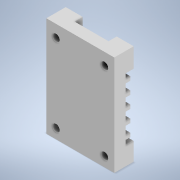
# Autodesk Inventor part: Belt Clamp
Saved by Autodesk Inventor 2020 (Build 240168000, 168)
## iProperties
Created: 2020-03-18
Part Number: Belt Clamp
Material: Generic
Document SubType Name: Modeling
Designer: DasNick
Density: 1 g/cm^3
Appearance: Default
Author: DasNick
Autodesk Inventor part; units mm, degrees
ref_plane "YZ Plane" through (0, 0, 0) normal (1, 0, 0) x (0, 1, 0)
ref_plane "XZ Plane" through (0, 0, 0) normal (0, 1, 0) x (-1, 0, 0)
sketch "Sketch1" plane through (0, 0, 0) normal (0, 0, 1) x (1, 0, 0)
  circle A0 centre (22.3624, 24.7247) radius 2.3813 projected
  circle A1 centre (22.3624, -26.3473) radius 2.3813 projected
  circle A2 centre (-9.3876, 24.7247) radius 2.3813 projected
  circle A3 centre (-9.3876, -26.3473) radius 2.3813 projected
  line L0 (28.7124, 32.6973) -> (-15.7376, 32.6973) projected
  line L1 (-15.7376, 32.6973) -> (-15.7376, -32.6973) projected
  line L2 (-15.7376, -32.6973) -> (28.7124, -32.6973) projected
  line L3 (28.7124, -32.6973) -> (28.7124, 32.6973) projected
  point P0 (0, 0)
extrude "Extrusion1" add sketch "Sketch1" along normal blind 12.7
sketch "Sketch2" plane through (-15.7376, -32.6973, 0) normal (0, -1, 0) x (1, 0, 0)
  line L0 (11.1075, 69.4178) -> (11.1075, 0)
  line L1 (33.3375, 69.1638) -> (33.3375, 0)
  line L2 (11.1075, 0) -> (33.3375, 0)
  line L3 (0, 9.525) -> (44.45, 9.525)
  line L4 (11.1075, 0) -> (33.3375, 0)
  line L5 (33.3375, 0) -> (33.3375, 5.334)
  line L6 (33.3375, 5.334) -> (11.1075, 5.334)
  line L7 (11.1075, 5.334) -> (11.1075, 0)
  line L8 (0, 0) -> (44.45, 0) projected
  point P0 (15.875, 0)
  point P1 (11.1075, 5.334)
  dimension "d2" = 5.334
  dimension "d21" = 0
  constraints: 16 end point, 1 point on line
  measures "d2" distance of L5.end L4.end
  measures "d21" distance between parallel lines of L8 L2
extrude "Extrusion2" cut sketch "Sketch2" against normal blind 76.2 contours L6 L1 L2 L0
ref_plane "Work Plane1" through (-16.0653, -32.8267, -33.655) normal (0, 0, -1) x (0, 1, 0)
sketch "Sketch3" plane through (17.5999, -32.6973, 5.334) normal (0, 0, -1) x (-1, 0, 0)
  line L0 (0, 0) -> (0, 65.3946) projected
  line L1 (0, 46.9796) -> (22.23, 46.9796)
  line L2 (22.23, 46.9796) -> (22.23, 49.5196)
  line L3 (22.23, 49.5196) -> (0, 49.5196)
  line L4 (0, 49.5196) -> (0, 46.9796)
  line L5 (0, 65.3946) -> (22.23, 65.3946) projected
  line L6 (33.3375, 65.3946) -> (33.3375, 0) projected
  line L7 (0, 38.9796) -> (22.23, 38.9796)
  line L8 (22.23, 38.9796) -> (22.23, 41.5196)
  line L9 (22.23, 41.5196) -> (0, 41.5196)
  line L10 (0, 41.5196) -> (0, 38.9796)
  line L11 (0, 30.9796) -> (22.23, 30.9796)
  line L12 (22.23, 30.9796) -> (22.23, 33.5196)
  line L13 (22.23, 33.5196) -> (0, 33.5196)
  line L14 (0, 33.5196) -> (0, 30.9796)
  line L15 (0, 22.9796) -> (22.23, 22.9796)
  line L16 (22.23, 22.9796) -> (22.23, 25.5196)
  line L17 (22.23, 25.5196) -> (0, 25.5196)
  line L18 (0, 25.5196) -> (0, 22.9796)
  line L19 (0, 14.9796) -> (22.23, 14.9796)
  line L20 (22.23, 14.9796) -> (22.23, 17.5196)
  line L21 (22.23, 17.5196) -> (0, 17.5196)
  line L22 (0, 17.5196) -> (0, 14.9796)
  point P0 (17.5999, 32.6973)
  point P1 (0, 17.5196)
  point P2 (0, 14.9796)
  point P3 (0, 25.5196)
  point P4 (0, 22.9796)
  point P5 (0, 33.5196)
  point P6 (0, 30.9796)
  point P7 (0, 41.5196)
  point P8 (0, 38.9796)
  point P9 (0, 49.5196)
  dimension "d6" = 15.875
  dimension "d7" = 2.54
  dimension "d10" = 8
  constraints: 40 end point, 2 parallel, 1 horizontal, 1 perpendicular, 1 point on line, 1 vertical, 32 other
  measures "d6" distance between parallel lines of L5 L3
  measures "d7" distance between parallel lines of L3 L1
  measures "d10" distance of L1.start L7.start
extrude "Extrusion3" add sketch "Sketch3" along normal blind 5.334
sketch "Sketch4" plane through (0, 0, 0) normal (0, 0, -1) x (-1, 0, 0)
  line L0 (4.6301, 14.2823) -> (4.6301, 16.8223)
  line L1 (15.7376, 32.6973) -> (15.7376, -32.6973) projected
  line L2 (4.6301, 16.8223) -> (15.7376, 16.8223)
  line L3 (15.7376, 16.8223) -> (15.7376, 19.9973)
  line L4 (15.7376, 19.9973) -> (4.6301, 19.9973)
  line L5 (4.6301, 19.9973) -> (4.6301, 16.8223)
  line L6 (4.6301, 14.2823) -> (4.6301, 8.8223)
  line L7 (4.6301, 6.2823) -> (4.6301, 0.8223)
  line L8 (4.6301, -1.7177) -> (4.6301, -7.1777)
  line L9 (4.6301, -9.7177) -> (4.6301, -15.1777)
  line L10 (-17.5999, 14.2823) -> (4.6301, 14.2823)
  line L11 (4.6301, 14.2823) -> (15.7376, 14.2823)
  line L12 (15.7376, 14.2823) -> (15.7376, 8.8223)
  line L13 (15.7376, 8.8223) -> (4.6301, 8.8223)
  line L14 (4.6301, 8.8223) -> (4.6301, 14.2823)
  line L15 (4.6301, 0.8223) -> (4.6301, 6.2823)
  line L16 (4.6301, 6.2823) -> (15.7376, 6.2823)
  line L17 (15.7376, 6.2823) -> (15.7376, 0.8223)
  line L18 (15.7376, 0.8223) -> (4.6301, 0.8223)
  line L19 (4.6301, 0.8223) -> (4.6301, 6.2823)
  line L20 (4.6301, -7.1777) -> (4.6301, -1.7177)
  line L21 (4.6301, -1.7177) -> (15.7376, -1.7177)
  line L22 (15.7376, -1.7177) -> (15.7376, -7.1777)
  line L23 (15.7376, -7.1777) -> (4.6301, -7.1777)
  line L24 (4.6301, -7.1777) -> (4.6301, -1.7177)
  line L25 (4.6301, -15.1777) -> (4.6301, -9.7177)
  line L26 (4.6301, -9.7177) -> (15.7376, -9.7177)
  line L27 (15.7376, -9.7177) -> (15.7376, -15.1777)
  line L28 (15.7376, -15.1777) -> (4.6301, -15.1777)
  line L29 (4.6301, -15.1777) -> (4.6301, -9.7177)
  line L30 (4.6301, -32.6973) -> (4.6301, -17.7177) projected
  line L31 (4.6301, -17.7177) -> (15.7376, -17.7177)
  line L32 (15.7376, -17.7177) -> (15.7376, -20.8927)
  line L33 (15.7376, -20.8927) -> (4.6301, -20.8927)
  line L34 (4.6301, -20.8927) -> (4.6301, -17.7177)
  line L35 (-28.7124, 32.6973) -> (15.7376, 32.6973) construction
  line L36 (-6.4874, 32.6973) -> (-6.4874, -33.4306) construction
  line L37 (-14.4, 16.8223) -> (-31.2231, 16.8223)
  line L38 (-31.2231, 16.8223) -> (-31.2231, 19.9973)
  line L39 (-31.2231, 19.9973) -> (-14.4, 19.9973)
  line L40 (-14.4, 19.9973) -> (-14.4, 16.8223)
  line L41 (-15.2764, -1.7177) -> (-15.2764, -7.1777)
  line L42 (-15.4955, -9.7177) -> (-15.4955, -15.1777)
  line L43 (-14.1435, 14.2823) -> (-30.6935, 14.2823)
  line L44 (-30.6935, 14.2823) -> (-30.6935, 8.8223)
  line L45 (-30.6935, 8.8223) -> (-16.0059, 8.8223)
  line L46 (-16.0059, 8.8223) -> (-14.1435, 14.2823)
  line L47 (-10.7606, 6.2823) -> (-30.4287, 6.2823)
  line L48 (-30.4287, 6.2823) -> (-30.4287, 0.8223)
  line L49 (-30.4287, 0.8223) -> (-15.6598, 0.8223)
  line L50 (-15.6598, 0.8223) -> (-10.7606, 6.2823)
  line L51 (-15.2764, -7.1777) -> (-15.2764, -1.7177)
  line L52 (-15.2764, -1.7177) -> (-29.0132, -1.7177)
  line L53 (-29.0132, -1.7177) -> (-29.0132, -7.1777)
  line L54 (-29.0132, -7.1777) -> (-15.2764, -7.1777)
  line L55 (-15.2764, -7.1777) -> (-15.2764, -1.7177)
  line L56 (-15.4955, -15.1777) -> (-15.4955, -9.7177)
  line L57 (-15.4955, -9.7177) -> (-29.8897, -9.7177)
  line L58 (-29.8897, -9.7177) -> (-29.8897, -15.1777)
  line L59 (-29.8897, -15.1777) -> (-15.4955, -15.1777)
  line L60 (-15.4955, -15.1777) -> (-15.4955, -9.7177)
  line L61 (-15.5503, -17.7177) -> (-32.0838, -17.7177)
  line L62 (-32.0838, -17.7177) -> (-32.0838, -20.8927)
  line L63 (-32.0838, -20.8927) -> (-15.5503, -20.8927)
  line L64 (-15.5503, -20.8927) -> (-15.5503, -17.7177)
  point P0 (0, 0)
  point P1 (-15.4955, -15.1777)
  point P2 (-15.2764, -7.1777)
  point P3 (4.6301, -20.8927)
  point P4 (15.7376, -17.7177)
  point P5 (4.6301, -15.1777)
  point P6 (15.7376, -9.7177)
  point P7 (15.7376, -1.7177)
  point P8 (4.6301, 0.8223)
  point P9 (15.7376, 6.2823)
  point P10 (4.6301, 8.8223)
  point P11 (15.7376, 14.2823)
  point P12 (15.7376, 16.8223)
  dimension "d17" = 3.175
  dimension "d18" = 3.175
  constraints: 126 end point, 6 point on line, 1 midpoint, 1 vertical
  measures "d17" distance of L3.end L2.end
  measures "d18" distance of L31.end L32.end
extrude "Extrusion4" cut sketch "Sketch4" against normal blind 5.334 contours L1 L33 L30 L31 | L1 L28 L9 L26 | L1 L23 L8 L21 | L1 L18 L7 L16 | L11 L1 L13 L6 | L46 L45 L44 L43 L10 | L5 L4 L1 L2 | L37 L38 L39 L40 | L41 L54 L53 L52 | L42 L59 L58 L57 | L50 L49 L48 L47 | L64 L63 L62 L61
sketch "Sketch5" plane through (0, 0, 0) normal (0, 0, -1) x (-1, 0, 0)
  line L0 (17.6982, 19.0646) -> (-30.6897, 19.0646)
  line L1 (-30.6897, 19.0646) -> (-30.6897, -19.7169)
  line L2 (-30.6897, -19.7169) -> (17.6982, -19.7169)
  line L3 (17.6982, -19.7169) -> (17.6982, 19.0646)
  constraints: 8 end point, 2 parallel, 1 horizontal, 1 perpendicular
extrude "Extrusion5" cut sketch "Sketch5" against normal blind 2.159
body "Solid1"
